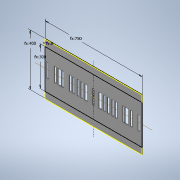
# Autodesk Inventor part: ferrite_layer_dex_1R1
Saved by Autodesk Inventor 2021 (Build 250183000, 183)
## iProperties
Created: 2021-01-27
Part Number: ferrite_layer_dex_1R1
Material: Generic
Document SubType Name: Modeling
Designer: pduy110
Density: 1 g/cm^3
Appearance: Smooth - Medium Gray
track_length: 750.000 mm
track_width: 300.000 mm
Author: pduy110
Autodesk Inventor part; units mm, degrees
ref_plane "YZ Plane" through (0, 0, 0) normal (1, 0, 0) x (0, 1, 0)
ref_plane "XZ Plane" through (0, 0, 0) normal (0, 1, 0) x (-1, 0, 0)
ref_plane "XY Plane" through (0, 0, 0) normal (0, 0, 1) x (1, 0, 0)
sketch "ferrite_layer_outline_sketch" plane through (0, 0, 0) normal (0, 0, 1) x (1, 0, 0)
  line L0 (-375, 200) -> (375, 200)
  line L1 (375, 200) -> (375, -200)
  line L2 (375, -200) -> (-375, -200)
  line L3 (-375, -200) -> (-375, 200)
  line L4 (0, 200) -> (0, -200) construction
  line L5 (0, 136.1953) -> (0, -273.5408) construction
  line L6 (0, 200) -> (0, -200)
  point P0 (0, 0)
  point P1 (0, 0)
  point P2 (0, 0)
  dimension "d85" = 750
  dimension "d86" = 400
  constraints: 14 end point, 4 midpoint, 2 parallel, 2 point on line, 1 coincident, 1 collinear, 1 horizontal, 1 perpendicular
  measures "d85" distance between parallel lines of L1 L3
  measures "d86" distance between parallel lines of L2 L0
extrude "Sheet Extrude" add sketch "ferrite_layer_outline_sketch" along normal blind 4
ref_plane "acrylic_sheet_plane" through (0, 0, 4) normal (0, 0, 1) x (1, 0, 0)
sketch "Sketch4" plane through (0, 0, 4) normal (0, 0, 1) x (1, 0, 0)
  line L0 (-360.5, 54.5) -> (-345.5, 54.5)
  line L1 (-345.5, 54.5) -> (-345.5, -54.5)
  line L2 (-345.5, -54.5) -> (-360.5, -54.5)
  line L3 (-360.5, -54.5) -> (-360.5, 54.5)
  line L4 (-12.6534, 0) -> (47.471, 0)
  line L5 (-375, 200) -> (-375, -200) projected
  line L6 (375, 200) -> (-375, 200) projected
  line L7 (-375, -200) -> (375, -200) projected
  point P0 (0, 0)
  point P1 (-360.5, 0)
  point P2 (-375, 0)
  dimension "d43" = 15
  dimension "d44" = 109
  dimension "d45" = 14.5
  constraints: 10 end point, 2 horizontal, 2 parallel, 2 point on line, 1 midpoint, 1 perpendicular, 2 other
  measures "d43" distance between parallel lines of L1 L3
  measures "d44" distance between parallel lines of L2 L0
extrude "Extrusion9" cut sketch "Sketch4" against normal through all
pattern_linear "Rectangular Pattern 7 fer" count 7 spacing 117.6667 along (1, 0, 0) of "Extrusion9"
pattern_linear "Rectangular Pattern 8 fer" count 8 spacing 100.8571 along (1, 0, 0) of "Extrusion9"
pattern_linear "pattern_test_#_of_ferrites 9 fer" count 9 spacing 88.25 along (1, 0, 0) of "Extrusion9"
pattern_linear "Rectangular Pattern 10 fer" [suppressed]
pattern_linear "Rectangular Pattern 13" count 13 spacing 58.8333 along (1, 0, 0) of "Extrusion9"
sketch "Sketch5" plane through (0, 0, 4) normal (0, 0, 1) x (1, 0, 0)
  line L0 (-375, 200) -> (-375, -200) projected
  line L1 (375, -200) -> (375, 200) projected
  line L2 (375, 200) -> (-375, 200) projected
  line L3 (-375, -200) -> (375, -200) projected
  line L4 (-375, 150) -> (375, 150)
  line L5 (375, 150) -> (375, -150)
  line L6 (375, -150) -> (-375, -150)
  line L7 (-375, -150) -> (-375, 150)
  line L8 (0, 150) -> (0, -150) construction
  line L9 (-375, 200) -> (-375, -200) construction
  circle A0 centre (-359.2579, 182.7315) radius 4
  point P0 (0, 0)
  dimension "d87" = 300
  dimension "d88" = 8
  constraints: 10 end point, 3 midpoint, 2 parallel, 1 centre point, 1 collinear, 1 horizontal, 1 perpendicular, 1 other
  measures "d87" distance between parallel lines of L6 L4
  measures "d88" diameter of A0
equation "\"d85\" = track_length"
equation "\"d86\" = layer_width"
equation "\"d43\" = ferrite_width"
equation "\"d44\" = ferrite_length"
equation "\"d45\" = edge_gap_distance"
equation "\"d50\" = parameter_5"
equation "\"d62\" = test_parameter_5"
equation "\"d87\" = track_width"
equation "\"d88\" = bolt_diameter"
equation "\"track_length\" = 750"
equation "\"track_width\" = 300"
equation "\"edge_gap_distance\" = 14.5"
equation "\"ferrite_length\" = 109"
equation "\"ferrite_width\" = 15"
equation "\"acrylic_sheet_8mm\" = 8"
equation "\"layer_width\" = 400"
equation "\"bolt_diameter\" = 8"
equation "\"ferrite_height\" = 8"
equation "\"y_offset_for_bolts\" = 175"
equation "\"wire_diameter\" = 4.5"
equation "\"distance_between_wires\" = -1.2 * wire_diameter + 0.2 * parameter_6"
equation "\"distance_between_wires_edge\" = -1.5 * wire_diameter + 0.5 * parameter_2"
equation "\"bend_radius_inner\" = 15"
equation "\"wall_thickness\" = 25"
equation "\"parameter_5\" = 117.666667"
equation "\"test_parameter_5\" = 88.25"
equation "\"parameter_6\" = 120"
equation "\"parameter_2\" = 30"
body "Solid8"
